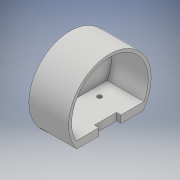
# Autodesk Inventor part: turn1part
Saved by Autodesk Inventor 2018 (Build 220112000, 112)
## iProperties
Created: 2019-10-09
Part Number: turn1part
Material: 一般
Document SubType Name: Modeling
Designer: Eiji Nishizawa
Density: 1 g/cm^3
Appearance: 既定
Author: Eiji Nishizawa
Autodesk Inventor part; units mm, degrees
ref_plane "YZ Plane" through (0, 0, 0) normal (1, 0, 0) x (0, 1, 0)
ref_plane "XZ Plane" through (0, 0, 0) normal (0, 1, 0) x (-1, 0, 0)
ref_plane "XY Plane" through (0, 0, 0) normal (0, 0, 1) x (1, 0, 0)
sketch "スケッチ1" plane through (0, 0, 0) normal (1, 0, 0) x (0, 1, 0)
  circle A0 centre (0, 0) radius 28
  circle A1 centre (0, 0) radius 8
  dimension "d0" = 56
  dimension "d1" = 16
  constraints: 2 centre point, 2 coincident
  measures "d0" diameter of A0
  measures "d1" diameter of A1
extrude "押し出し1" add sketch "スケッチ1" along normal blind 2
sketch "スケッチ2" plane through (2, 0, 0) normal (1, 0, 0) x (0, 0, -1)
  circle A0 centre (0, 0) radius 28 projected
  line L0 (16.6658, 22.5) -> (16.6658, -22.5)
  line L1 (14.6658, -24.1923) -> (14.6658, 23.8519)
  arc A1 (16.6658, 22.5) -> (14.6658, 23.8519) centre (0, 0) ccw
  arc A2 (14.6038, -23.89) -> (16.6658, -22.5) centre (0, 0) ccw
  arc A3 (14.6658, 23.8519) -> (14.6038, -23.89) centre (0, 0) ccw
  arc A4 (14.6658, 21.4689) -> (14.5463, -21.5501) centre (0, 0) ccw
  dimension "d4" = 2
  dimension "d30" = 45
  dimension "d31" = 2
  constraints: 10 point on circle, 4 centre point, 4 coincident, 4 end point, 2 vertical, 1 point on line
  measures "d4" radial gap between concentric circles of A0 A4
  measures "d30" distance of L0.start L0.end
  measures "d31" distance between parallel lines of L0 L1
extrude "押し出し2" add sketch "スケッチ2" along normal blind 25 contours L0 A0 L1 | L1 A0
sketch "スケッチ3" plane through (27, 0, 0) normal (1, 0, 0) x (0, 0, -1)
  circle A0 centre (0, 0) radius 28 projected
  line L0 (16.6658, -22.5) -> (16.6658, 22.5) projected
  line L1 (16.6658, 22.5) -> (16.6658, -22.5)
  arc A1 (16.6658, 22.5) -> (16.6658, -22.5) centre (0, 0) ccw
  arc A2 (16.6658, 19.9562) -> (16.6658, -19.9562) centre (0, 0) ccw
  line L2 (11.6658, -23.2359) -> (11.6658, 23.2359)
  dimension "d7" = 2
  dimension "d8" = 5
  constraints: 7 point on circle, 4 end point, 2 centre point, 2 coincident, 2 point on line, 1 collinear, 1 vertical
  measures "d7" radial gap between concentric circles of A0 A2
  measures "d8" distance between parallel lines of L0 L2
extrude "押し出し3" cut sketch "スケッチ3" against normal blind 25 contours L2 A2
sketch "スケッチ4" plane through (2, -22.5, -16.6658) normal (0, 0, -1) x (-1, 0, 0)
  line L0 (-25, 0) -> (-25, 45) projected
  line L1 (-25, 30) -> (-22, 30)
  line L2 (-22, 30) -> (-22, 15)
  line L3 (-22, 15) -> (-25, 15)
  line L4 (-25, 15) -> (-25, 30)
  line L5 (0, 45) -> (-25, 45) projected
  line L6 (0, 0) -> (-25, 0) projected
  point P0 (2, 22.5)
  dimension "d11" = 15
  dimension "d12" = 15
  dimension "d13" = 3
  constraints: 8 end point, 2 parallel, 1 horizontal, 1 perpendicular, 1 point on line
  measures "d11" distance between parallel lines of L5 L1
  measures "d12" distance between parallel lines of L6 L3
  measures "d13" distance of L2.end L3.end
extrude "押し出し4" cut sketch "スケッチ4" against normal blind 25
sketch "スケッチ5" plane through (2, -22.5, -16.6658) normal (0, 0, -1) x (-1, 0, 0)
  circle A0 centre (-7, 11.5) radius 1.5
  circle A1 centre (-7, 33.5) radius 1.5
  line L0 (-13, 7.5) -> (-1, 7.5)
  line L1 (-1, 7.5) -> (-1, 37.5)
  line L2 (-1, 37.5) -> (-13, 37.5)
  line L3 (-13, 37.5) -> (-13, 7.5)
  line L4 (0, 45) -> (0, 0) projected
  line L5 (0, 45) -> (-25, 45) projected
  line L6 (0, 0) -> (-25, 0) projected
  point P0 (2, 22.5)
  dimension "d16" = 3
  dimension "d17" = 3
  dimension "d19" = 30
  dimension "d20" = 4
  dimension "d21" = 4
  dimension "d22" = 6
  dimension "d23" = 6
  dimension "d24" = 6
  dimension "d25" = 1
  dimension "d26" = 7.5
  dimension "d27" = 7.5
  constraints: 8 end point, 2 centre point, 2 parallel, 1 horizontal, 1 perpendicular
  measures "d16" diameter of A0
  measures "d17" diameter of A1
  measures "d19" distance of L2.end L0.start
  measures "d20" distance from line of L0 A0.centre
  measures "d21" distance from line of L2 A1.centre
  measures "d22" distance from line of L3 A0.centre
  measures "d23" distance from line of L1 A0.centre
  measures "d24" distance from line of L1 A1.centre
  measures "d25" distance between parallel lines of L4 L1
  measures "d26" distance between parallel lines of L5 L2
  measures "d27" distance between parallel lines of L6 L0
extrude "押し出し5" cut sketch "スケッチ5" against normal blind 25 contours A0 | A1
sketch "スケッチ6" plane through (2, -22.5, -16.6658) normal (0, 0, -1) x (-1, 0, 0)
  point P0 (2, 22.5)
